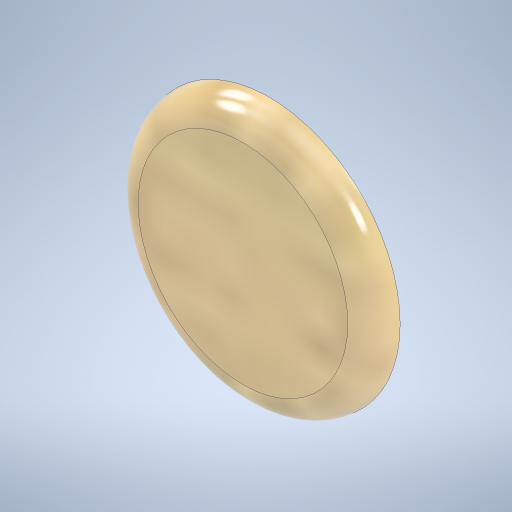
# Autodesk Inventor part: Cap
Saved by Autodesk Inventor 2024 (Build 280153000, 153)
## iProperties
Created: 2021-05-10
Part Number: Cap
Material: Generic
Document SubType Name: Modeling
Designer: RokasM
Density: 1 g/cm^3
Appearance: Default
Author: RokasM
Autodesk Inventor part; units mm, degrees
ref_plane "YZ Plane" through (0, 0, 0) normal (1, 0, 0) x (0, 1, 0)
ref_plane "XZ Plane" through (0, 0, 0) normal (0, 1, 0) x (-1, 0, 0)
ref_plane "XY Plane" through (0, 0, 0) normal (0, 0, 1) x (1, 0, 0)
sketch "Sketch1" plane through (0, 0, 0) normal (0, 0, 1) x (1, 0, 0)
  circle A0 centre (0, 0) radius 5 projected
extrude "Extrusion1" add sketch "Sketch1" along normal blind 1
fillet "Fillet1" radius 1 1 edges at (-5, 0, 1)
